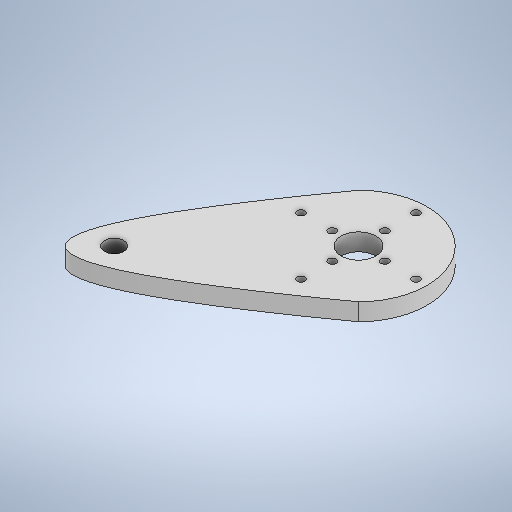
# Autodesk Inventor part: Servo-head.finalV1
Saved by Autodesk Inventor 2025.2 (Build 292293000, 293)
## iProperties
Created: 2025-04-29
Part Number: Servo-head.finalV1
Material: Generic
Document SubType Name: Modeling
Designer: patrickandersen
Density: 1 g/cm^3
Appearance: Default
Author: patrickandersen
Autodesk Inventor part; units mm, degrees
ref_plane "YZ Plane" through (0, 0, 0) normal (1, 0, 0) x (0, 1, 0)
ref_plane "XZ Plane" through (0, 0, 0) normal (0, 1, 0) x (-1, 0, 0)
ref_plane "XY Plane" through (0, 0, 0) normal (0, 0, 1) x (1, 0, 0)
sketch "Sketch1" plane through (0, 0, 0) normal (0, 1, 0) x (-1, 0, 0)
  circle A0 centre (0, 0) radius 19.75
  circle A1 centre (0, 0) radius 5
  circle A2 centre (0, 16.6) radius 1.1
  circle A3 centre (16.6, 0) radius 1.1
  circle A4 centre (0, -16.6) radius 1.1
  circle A5 centre (-16.6, 0) radius 1.1
  circle A6 centre (-7.6, 0) radius 1.1
  circle A7 centre (0, 7.6) radius 1.1
  circle A8 centre (7.6, 0) radius 1.1
  circle A9 centre (0, -7.6) radius 1.1
  point P0 (0, 19.75)
  point P1 (19.75, 0)
  point P2 (0, -19.75)
  point P3 (-19.75, 0)
  point P4 (0, -5)
  point P5 (-5, 0)
  point P6 (0, 5)
  point P7 (5, 0)
  dimension "d0" = 39.5
  dimension "d1" = 10
  dimension "d2" = 2.2
  dimension "d3" = 3.15
  dimension "d4" = 2.2
  dimension "d5" = 3.15
  dimension "d6" = 2.2
  dimension "d7" = 3.15
  dimension "d8" = 2.2
  dimension "d9" = 3.15
  dimension "d10" = 2.2
  dimension "d11" = 2.2
  dimension "d12" = 2.2
  dimension "d13" = 2.2
  dimension "d14" = 2.6
  dimension "d15" = 2.6
  dimension "d16" = 2.6
  dimension "d17" = 2.6
  constraints: 10 centre point, 8 point on circle, 2 coincident
  measures "d0" diameter of A0
  measures "d1" diameter of A1
  measures "d2" diameter of A2
  measures "d3" distance of A0.start A2.centre
  measures "d4" diameter of A3
  measures "d5" distance of A3.centre A0.end
  measures "d6" diameter of A4
  measures "d7" distance of point (0, -19.75) A4.centre
  measures "d8" diameter of A5
  measures "d9" distance of point (-19.75, 0) A5.centre
  measures "d10" diameter of A6
  measures "d11" diameter of A7
  measures "d12" diameter of A8
  measures "d13" diameter of A9
  measures "d14" distance of point (5, 0) A8.centre
  measures "d15" distance of point (0, 5) A7.centre
  measures "d16" distance of A1.start A9.centre
  measures "d17" distance of A1.end A6.centre
extrude "Extrusion1" add sketch "Sketch1" along normal blind 5
sketch "Sketch2" plane through (0, 5, 0) normal (0, 1, 0) x (1, 0, 0)
  line L0 (17.6777, 17.6777) -> (67.6777, 17.6777) construction
  line L1 (0, 0) -> (-35.3553, -35.3553)
  line L2 (0, 0) -> (50, 0) construction
  circle A0 centre (-35.3553, -35.3553) radius 2.75
  circle A1 centre (0, 0) radius 19.75 projected
  line L3 (13.9654, -13.9654) -> (-13.9654, 13.9654)
  line L4 (-13.9654, 13.9654) -> (-56.3918, -28.461)
  line L5 (13.9654, -13.9654) -> (-28.461, -56.3918)
  line L6 (-28.461, -56.3918) -> (-56.3918, -28.461)
  circle A2 centre (0, -16.6) radius 1.1 projected
  circle A3 centre (0, -16.6) radius 1.1
  circle A4 centre (0, -7.6) radius 1.1 projected
  circle A5 centre (0, -7.6) radius 1.1
  circle A6 centre (-7.6, 0) radius 1.1 projected
  circle A7 centre (-7.6, 0) radius 1.1
  circle A8 centre (-16.6, 0) radius 1.1 projected
  circle A9 centre (-16.6, 0) radius 1.1
  circle A10 centre (0, 0) radius 5
  dimension "d22" = 50
  dimension "d23" = 135
  dimension "d24" = 5.5
  dimension "d25" = 60
  dimension "d26" = 60
  constraints: 14 end point, 6 centre point, 6 coincident, 2 horizontal, 2 perpendicular, 2 point on circle, 1 equal length, 1 tangent
  measures "d22" distance of L1.start L1.end
  measures "d23" angle of L1 L2
  measures "d24" diameter of A0
  measures "d25" distance of L3.end L4.end
  measures "d26" distance of L3.start L5.end
extrude "Extrusion2" add sketch "Sketch2" against normal blind 5 contours A1 L5 L6 L4
sketch "Sketch3" plane through (0, 5, 0) normal (0, 1, 0) x (1, 0, 0)
  line L0 (-28.461, -56.3918) -> (-56.3918, -28.461) projected
  arc A0 (13.9654, -13.9654) -> (-13.9654, 13.9654) centre (0, 0) ccw projected
  line L1 (-28.461, -56.3918) -> (13.9654, -13.9654) projected
  spline S0 degree 2 poles (-13.9654, 13.9654) (-84.8528, -84.8528) (13.9654, -13.9654) knots 0 0 0 1 1 1
  line L2 (13.9654, -13.9654) -> (-28.461, -56.3918)
  line L3 (-56.3918, -28.461) -> (-13.9654, 13.9654)
  point P0 (-42.4264, -42.4264)
  constraints: 4 end point, 2 equal length, 1 midpoint, 3 other
extrude "Extrusion3" cut sketch "Sketch3" against normal blind 5 contours L0 S0 L1 | L0 L3 S0
body "Solid1"
